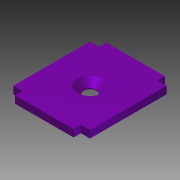
# Autodesk Inventor part: 13_0204_042
Saved by Autodesk Inventor 2012 SP1 (Build 160190100, 190)
## iProperties
Created: 2013-04-08
Part Number: 13_0204_042
Material: Default
Document SubType Name: Modeling
Designer: vogel
Density: 1 g/cm^3
Author: vogel
Autodesk Inventor part; units mm, degrees
ref_plane "YZ Plane" through (0, 0, 0) normal (1, 0, 0) x (0, 1, 0)
ref_plane "XZ Plane" through (0, 0, 0) normal (0, 1, 0) x (-1, 0, 0)
ref_plane "XY Plane" through (0, 0, 0) normal (0, 0, 1) x (1, 0, 0)
sketch "Skizze1" plane through (0, 0, 0) normal (0, 0, 1) x (1, 0, 0)
  line L0 (-14.7, 0) -> (14.7, 0) projected
  line L1 (0, -17.5) -> (0, 17.5) projected
  line L2 (10.5, 10.5) -> (10.5, -10.5)
  line L3 (-10.5, -10.5) -> (-10.5, 10.5)
  line L4 (8, 10.5) -> (8, 12.5)
  line L5 (8, 12.5) -> (-8, 12.5)
  line L6 (-8, 12.5) -> (-8, 10.5)
  line L7 (8, -10.5) -> (8, -12.5)
  line L8 (8, -12.5) -> (-8, -12.5)
  line L9 (-8, -12.5) -> (-8, -10.5)
  line L10 (-10.5, 10.5) -> (-8, 10.5)
  line L11 (8, 10.5) -> (10.5, 10.5)
  line L12 (10.5, -10.5) -> (8, -10.5)
  line L13 (-8, -10.5) -> (-10.5, -10.5)
  point P0 (0, 0)
  dimension "d0" = 21
  dimension "d1" = 21
  dimension "d2" = 25
  dimension "d3" = 16
  constraints: 24 end point, 7 parallel, 3 collinear, 2 horizontal, 2 perpendicular, 5 other
  measures "d0" distance between parallel lines of L2 L3
  measures "d1" distance between parallel lines of L13 L10
  measures "d2" distance between parallel lines of L8 L5
  measures "d3" distance between parallel lines of L4 L6
extrude "Extrusion1" add sketch "Skizze1" along normal blind 2
sketch "Skizze2" plane through (0, 0, 2) normal (0, 0, 1) x (1, 0, 0)
  point P0 (0, 0)
  point P1 (0, 0)
  constraints: 1 coincident
hole "Bohrung1" at (0, 0, 2) direction (0, 0, -1) diameter 3.4 end through all countersink diameter 6.9 countersink angle 90
